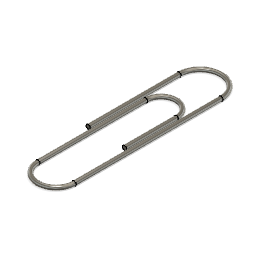
Day #3 - Paper Clip v2 (Autodesk Fusion 360 design; units mm, degrees)
Autodesk Fusion 360 part; units mm, degrees
sketch "Sketch1" plane through (0, 0, 0) normal (0, 1, 0) x (1, 0, 0) in component "Clip"
  line L0 (0, 0) -> (0, 16.25)
  line L1 (0, 0) -> (7.5, 0) construction
  line L2 (7.5, 0) -> (7.5, 16.25)
  line L3 (7.5, 0) -> (7.5, -10)
  line L4 (7.5, -10) -> (1, -10) construction
  line L5 (1, -10) -> (1, 9.25)
  line L6 (1, 9.25) -> (6.5, 9.25) construction
  line L7 (6.5, 9.25) -> (6.5, 0)
  line L8 (0, 16.25) -> (7.5, 16.25) construction
  arc A0 (7.5, 16.25) -> (0, 16.25) centre (3.75, 16.25) ccw
  arc A1 (1, -10) -> (7.5, -10) centre (4.25, -10) ccw
  arc A2 (6.5, 9.25) -> (1, 9.25) centre (3.75, 9.25) ccw
  dimension "d1" = 16.25
  dimension "d2" = 7.5
  dimension "d5" = 6.5
  dimension "d6" = 19.25
  dimension "d7" = 5.5
  dimension "d8" = 26.25
  constraint coincident L0.start L1.start
  constraint vertical L0
  constraint perpendicular L0 L1
  constraint perpendicular L1 L2
  constraint perpendicular L1 L3
  constraint perpendicular L3 L4
  constraint perpendicular L1 L5
  constraint perpendicular L5 L6
  constraint coincident L1 L7.end
  constraint perpendicular L1 L7
  constraint perpendicular L2 L8
  constraint tangent L0 A0
  constraint tangent L5 A1
  constraint tangent L5 A2
  measures "d1" distance of L0.start L0.end
  measures "d2" distance of L0.start L1.end
  measures "d5" distance of L3.end L4.end
  measures "d6" distance of L4.end L5.end
  measures "d7" distance of L5.end L6.end
  measures "d8" distance of L2.end L3.end
sketch "Sketch2" plane through (0, 0, 0) normal (0, 0, 1) x (1, 0, 0) in component "Clip"
  circle A0 centre (0, 0) radius 0.375
  dimension "d9" = 0.75
  constraint coincident A0.centre origin
  measures "d9" diameter of A0
sweep "Sweep1" add profiles "Sketch2" path "Sketch1" along L0 A0 L2 L3 A1 L5 A2 L7 section 1 in component "Clip"
component "Clip" placed x (1, 0, 0) y (0, 1, 0) z (0, 0, 1) at (0, 0, 0)
